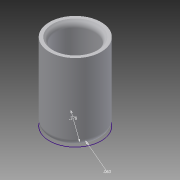
# Autodesk Inventor part: 137 V Dipole Cap
Saved by Autodesk Inventor 2014 (Build 180170000, 170)
## iProperties
Created: 2023-07-11
Part Number: 137 V Dipole Cap
Material: Generic
Document SubType Name: Modeling
Designer: VMUser
Density: 1 g/cm^3
Appearance: Default
Author: VMUser
Autodesk Inventor part; units mm, degrees
ref_plane "YZ Plane" through (0, 0, 0) normal (1, 0, 0) x (0, 1, 0)
ref_plane "XZ Plane" through (0, 0, 0) normal (0, 1, 0) x (-1, 0, 0)
ref_plane "XY Plane" through (0, 0, 0) normal (0, 0, 1) x (1, 0, 0)
sketch "Sketch1" plane through (0, 0, 0) normal (0, 1, 0) x (-1, 0, 0)
  circle A0 centre (0, 0) radius 4.8006
  circle A1 centre (0, 0) radius 6.3881
  dimension "d0" = 9.6012
  dimension "d1" = 1.5875
  constraints: 2 centre point, 1 coincident
  measures "d0" diameter of A0
  measures "d1" radial gap between concentric circles of A1 A0
extrude "Extrusion1" add sketch "Sketch1" along normal blind 19.05
extrude "Extrusion2" add sketch "Sketch1" along normal blind 3.175 contours A0
fillet "Fillet1" radius 1.5875 1 edges at (6.3881, 0, 0)
chamfer "Chamfer1" distance 0.7937 angle 45 1 edges at (4.8006, 19.05, 0)
fillet "Fillet2" radius 1.5875 1 edges at (4.8006, 18.2563, 0)
body "Solid1"
